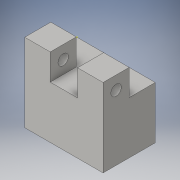
# Autodesk Inventor part: HingePart2MK2
Saved by Autodesk Inventor 2016 (Build 200138000, 138)
## iProperties
Created: 2017-02-18
Part Number: HingePart2MK2
Material: Generic
Document SubType Name: Modeling
Designer: RoboticsUser
Density: 1 g/cm^3
Appearance: Default
Author: RoboticsUser
Autodesk Inventor part; units mm, degrees
ref_plane "YZ Plane" through (0, 0, 0) normal (1, 0, 0) x (0, 1, 0)
ref_plane "XZ Plane" through (0, 0, 0) normal (0, 1, 0) x (-1, 0, 0)
ref_plane "XY Plane" through (0, 0, 0) normal (0, 0, 1) x (1, 0, 0)
sketch "Sketch1" plane through (0, 0, 0) normal (0, 0, 1) x (1, 0, 0)
  line L0 (0, 0) -> (9.525, 0)
  line L1 (9.525, 0) -> (9.525, 6.35)
  line L2 (9.525, 6.35) -> (0, 6.35)
  line L3 (0, 6.35) -> (0, 0)
  dimension "d0" = 9.525
  dimension "d1" = 6.35
  constraints: 8 end point, 2 parallel, 1 horizontal, 1 perpendicular
  measures "d0" distance of L2.end L1.end
  measures "d1" distance of L1.end L0.end
extrude "Extrusion1" add sketch "Sketch1" along normal blind 6.35
sketch "Sketch2" plane through (0, 6.35, 0) normal (0, 1, 0) x (1, 0, 0)
  point P0 (0, 0)
sketch "Sketch3" plane through (0, 6.35, 0) normal (0, 1, 0) x (1, 0, 0)
  line L0 (0, 0) -> (0, -6.35) projected
  line L1 (0, -6.35) -> (9.525, -6.35) projected
  line L2 (0, -3.175) -> (3.0988, -3.175)
  line L3 (3.0988, -3.175) -> (3.0988, -6.35)
  line L4 (3.0988, -6.35) -> (0, -6.35)
  line L5 (0, -6.35) -> (0, -3.175)
  dimension "d4" = 3.0988
  constraints: 8 end point, 2 parallel, 1 horizontal, 1 midpoint, 1 perpendicular, 1 point on line
  measures "d4" distance of L3.end L4.end
extrude "Extrusion2" add sketch "Sketch3" along normal blind 3.175
sketch "Sketch4" plane through (0, 6.35, 0) normal (0, 1, 0) x (1, 0, 0)
  line L0 (9.525, 0) -> (9.525, -6.35) projected
  line L1 (0, -6.35) -> (9.525, -6.35) projected
  line L2 (9.525, -3.175) -> (6.4262, -3.175)
  line L3 (6.4262, -3.175) -> (6.4262, -6.35)
  line L4 (6.4262, -6.35) -> (9.525, -6.35)
  line L5 (9.525, -6.35) -> (9.525, -3.175)
  point P0 (0, 0)
  dimension "d7" = 3.0988
  constraints: 8 end point, 2 parallel, 1 horizontal, 1 midpoint, 1 perpendicular, 1 point on line
  measures "d7" distance of L4.end L3.end
extrude "Extrusion3" add sketch "Sketch4" along normal blind 3.175
hole "Hole1" at (9.525, 7.9248, 4.7752) direction (-1, 0, 0) diameter 1.27 end through all
body "Solid1"
